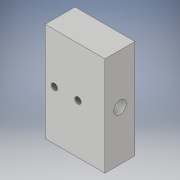
# Autodesk Inventor part: MotorMount
Saved by Autodesk Inventor 2019.3 (Build 233278000, 278)
## iProperties
Created: 2019-01-26
Part Number: MotorMount
Material: Generic
Document SubType Name: Modeling
Designer: mark
Density: 1 g/cm^3
Appearance: Default
Author: mark
Autodesk Inventor part; units mm, degrees
ref_plane "YZ Plane" through (0, 0, 0) normal (1, 0, 0) x (0, 1, 0)
ref_plane "XZ Plane" through (0, 0, 0) normal (0, 1, 0) x (-1, 0, 0)
ref_plane "XY Plane" through (0, 0, 0) normal (0, 0, 1) x (1, 0, 0)
sketch "Sketch1" plane through (0, 0, 0) normal (0, 0, 1) x (1, 0, 0)
  line L0 (0, 0) -> (76.2, 0)
  line L1 (76.2, 0) -> (76.2, 125.8)
  line L2 (76.2, 125.8) -> (0, 125.8)
  line L3 (0, 125.8) -> (0, 0)
  circle A0 centre (12, 62.9) radius 4
  circle A1 centre (42, 62.9) radius 4
  dimension "d0" = 76.2
  dimension "d1" = 125.8
  dimension "d2" = 8
  dimension "d3" = 8
  dimension "d4" = 12
  dimension "d5" = 42
  dimension "d6" = 62.9
  dimension "d7" = 62.9
  constraints: 8 end point, 2 centre point, 2 perpendicular, 1 horizontal
  measures "d0" distance of L2.end L1.end
  measures "d1" distance between parallel lines of L0 L2
  measures "d2" diameter of A0
  measures "d3" diameter of A1
  measures "d4" distance from line of L3 A0.centre
  measures "d5" distance from line of L3 A1.centre
  measures "d6" distance from line of L0 A1.centre
  measures "d7" distance from line of L0 A0.centre
extrude "Extrusion1" add sketch "Sketch1" along normal blind 38.2 contours L3 L2 L1 L0 | A0 | A1
sketch "Sketch2" plane through (0, 0, 38.2) normal (0, 0, 1) x (1, 0, 0)
  line L0 (0, 0) -> (76.2, 0)
  line L1 (76.2, 0) -> (76.2, 125.8)
  line L2 (76.2, 125.8) -> (0, 125.8)
  line L3 (0, 125.8) -> (0, 0)
  circle A0 centre (12, 62.9) radius 4
  circle A1 centre (42, 62.9) radius 4
  dimension "d17" = 76.2
  dimension "d16" = 125.8
  dimension "d13" = 8
  dimension "d10" = 8
  dimension "d15" = 12
  dimension "d12" = 42
  dimension "d11" = 62.9
  dimension "d14" = 62.9
  constraints: 8 end point, 2 centre point, 2 perpendicular, 1 horizontal
  measures "d17" distance of L2.end L1.end
  measures "d16" distance between parallel lines of L0 L2
  measures "d13" diameter of A0
  measures "d10" diameter of A1
  measures "d15" distance from line of L3 A0.centre
  measures "d12" distance from line of L3 A1.centre
  measures "d11" distance from line of L0 A1.centre
  measures "d14" distance from line of L0 A0.centre
extrude "Extrusion2" cut sketch "Sketch2" against normal blind 19.1 contours A0 | A1
sketch "Sketch3" plane through (0, 0, 0) normal (-1, 0, 0) x (0, 0, 1)
  circle A0 centre (19.1, 62.9) radius 8
  line L0 (38.2, 125.8) -> (38.2, 0) projected
  line L1 (0, 0) -> (38.2, 0) projected
  dimension "d21" = 16
  dimension "d22" = 19.1
  dimension "d23" = 62.9
  constraints: 1 centre point
  measures "d21" diameter of A0
  measures "d22" distance from line of L0 A0.centre
  measures "d23" distance from line of L1 A0.centre
extrude "Extrusion3" cut sketch "Sketch3" against normal up to next
thread "Thread1" size "M8x1.25" class "6H" standard "ANSI Metric M Profile" full length
thread "Thread2" size "M8x1.25" class "6H" standard "ANSI Metric M Profile" full length
body "Solid1"
